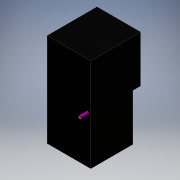
# Autodesk Inventor part: camera
Saved by Autodesk Inventor 2016 (Build 200138000, 138)
## iProperties
Created: 2015-10-17
Part Number: camera
Material: Generic
Document SubType Name: Modeling
Designer: Artur
Density: 1 g/cm^3
Appearance: Default
Mass: 48.6921 g
Surface Area: 89.5904 cm^2
Volume: 48.6921 cm^3
Author: Artur
Autodesk Inventor part; units mm, degrees
ref_plane "YZ Plane" through (0, 0, 0) normal (1, 0, 0) x (0, 1, 0)
ref_plane "XZ Plane" through (0, 0, 0) normal (0, 1, 0) x (-1, 0, 0)
ref_plane "XY Plane" through (0, 0, 0) normal (0, 0, 1) x (1, 0, 0)
sketch "Sketch1" plane through (0, 0, 0) normal (0, 1, 0) x (-1, 0, 0)
  line L0 (0, 0) -> (28, 0)
  line L1 (28, 0) -> (28, -60)
  line L2 (28, -60) -> (0, -60)
  line L3 (0, -60) -> (0, 0)
  dimension "d0" = 60
  dimension "d1" = 28
  constraints: 8 end point, 2 parallel, 1 horizontal, 1 perpendicular
  measures "d0" distance of L0.end L1.end
  measures "d1" distance of L1.end L2.end
extrude "Extrusion1" add sketch "Sketch1" along normal blind 27
sketch "Sketch2" plane through (0, 27, 0) normal (0, 1, 0) x (1, 0, 0)
  line L0 (0, 0) -> (0, 60) projected
  line L1 (0, 0) -> (-28, 0)
  line L2 (-28, 0) -> (-28, 30)
  line L3 (-28, 30) -> (0, 30)
  line L4 (0, 30) -> (0, 0)
  line L5 (-28, 60) -> (-28, 0) projected
  dimension "d4" = 30
  constraints: 8 end point, 2 parallel, 1 collinear, 1 horizontal, 1 perpendicular
  measures "d4" distance of L1.end L2.end
extrude "Extrusion2" add sketch "Sketch2" along normal blind 5
sketch "Sketch3" plane through (0, 32, 0) normal (0, 1, 0) x (1, 0, 0)
  circle A0 centre (-14, 15) radius 7.5
  line L0 (0, 30) -> (-28, 30) construction
  line L1 (-28, 0) -> (0, 0) construction
  line L2 (0, 0) -> (0, 30) construction
  line L3 (0, 30) -> (-28, 30) construction
  line L4 (-28, 30) -> (-28, 0) construction
  line L5 (-28, 0) -> (0, 0) construction
  line L6 (-28, 30) -> (-28, 0) construction
  line L7 (-14, 0) -> (-14, 30) construction
  line L8 (-28, 15) -> (0, 15) construction
  line L9 (0, 60) -> (0, 0) construction
  point P0 (-14, 15)
  point P1 (-14, 15)
  dimension "d7" = 15
  constraints: 5 midpoint, 4 end point, 1 centre point, 1 coincident, 1 perpendicular, 1 point on line
  measures "d7" diameter of A0
extrude "Extrusion3" cut sketch "Sketch3" against normal blind 5
sketch "Sketch4" plane through (0, 0, 0) normal (0, -1, 0) x (1, 0, 0)
  circle A0 centre (-2, -30) radius 1
  line L0 (0, -60) -> (0, 0) projected
  line L1 (0, -30) -> (0, -60) projected
  line L2 (0, -30) -> (-52.148, -30)
  line L3 (0, -30) -> (-28, -30) projected
  dimension "d10" = 2
  dimension "d11" = 2
  constraints: 2 end point, 1 centre point, 1 collinear, 1 point on line
  measures "d10" diameter of A0
  measures "d11" distance from line of L0 A0.centre
extrude "Extrusion4" add sketch "Sketch4" along normal blind 5
sketch "Sketch5" plane through (-2, -5, -30) normal (0, -1, 0) x (1, 0, 0)
  circle A0 centre (0, 0) radius 1 projected
  point P0 (2, 30)
  constraints: 1 coincident
body "Solid1"
